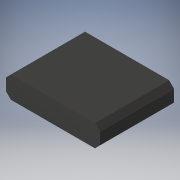
# Autodesk Inventor part: NESE 2S2P
Saved by Autodesk Inventor 2019.2 (Build 232265000, 265)
## iProperties
Created: 2019-05-20
Part Number: NESE 2S2P
Material: Generic
Document SubType Name: Modeling
Designer: Johansson
Density: 1 g/cm^3
Appearance: Default
Author: Johansson
Autodesk Inventor part; units mm, degrees
ref_plane "YZ Plane" through (0, 0, 0) normal (1, 0, 0) x (0, 1, 0)
ref_plane "XZ Plane" through (0, 0, 0) normal (0, 1, 0) x (-1, 0, 0)
ref_plane "XY Plane" through (0, 0, 0) normal (0, 0, 1) x (1, 0, 0)
sketch "Sketch1" plane through (0, 0, 0) normal (0, 1, 0) x (-1, 0, 0)
  line L0 (-47.5, 37.5) -> (47.5, 37.5)
  line L1 (47.5, 37.5) -> (47.5, -37.5)
  line L2 (47.5, -37.5) -> (-47.5, -37.5)
  line L3 (-47.5, -37.5) -> (-47.5, 37.5)
  line L4 (-47.5, 37.5) -> (47.5, -37.5) construction
  line L5 (47.5, 37.5) -> (-47.5, -37.5) construction
  point P0 (0, 0)
  dimension "d0" = 95
  dimension "d1" = 75
  constraints: 12 end point, 2 midpoint, 2 parallel, 1 horizontal, 1 perpendicular
  measures "d0" distance between parallel lines of L3 L1
  measures "d1" distance of L0.end L1.end
extrude "Extrusion1" add sketch "Sketch1" along normal blind 22
chamfer "Chamfer1" distance 5 angle 45 4 edges at (-47.5, 22, 0) (47.5, 22, 0) (47.5, 0, 0) (-47.5, 0, 0)
body "Solid1"
